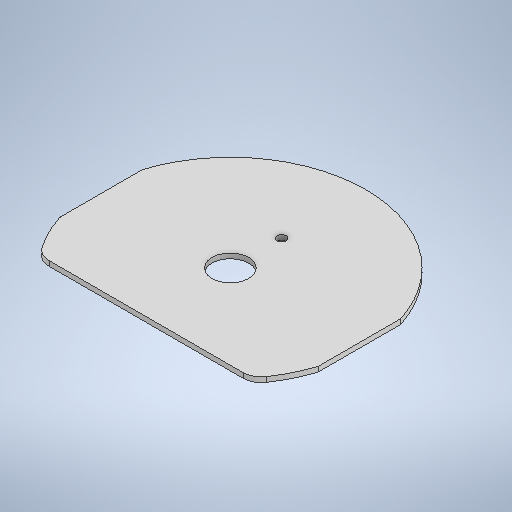
# Autodesk Inventor part: tapa_carcasa_4.0
Saved by Autodesk Inventor 2025.3 (Build 293356030, 356C)
## iProperties
Created: 2025-10-09
Part Number: tapa_carcasa_4.0
Material: Generic
Document SubType Name: Modeling
Designer: brene
Density: 1 g/cm^3
Appearance: Default
Author: brene
Autodesk Inventor part; units mm, degrees
ref_plane "YZ Plane" through (0, 0, 0) normal (1, 0, 0) x (0, 1, 0)
ref_plane "XZ Plane" through (0, 0, 0) normal (0, 1, 0) x (-1, 0, 0)
ref_plane "XY Plane" through (0, 0, 0) normal (0, 0, 1) x (1, 0, 0)
sketch "Sketch3" plane through (0, 0, 0) normal (0, 1, 0) x (-1, 0, 0)
  line L0 (0, 0) -> (67.5, 0)
  line L1 (0, 0) -> (0, 46)
  line L2 (70.5, 22.4889) -> (70.5, -22.4889)
  line L3 (0, 46) -> (52.915, 46)
  line L4 (-70.5, 22.4889) -> (-70.5, -22.4889)
  line L5 (0, 46) -> (-52.915, 46)
  arc A0 (70.5, 22.4889) -> (61.183, 41.625) centre (0, 0) ccw
  arc A1 (-61.183, 41.625) -> (-70.5, 22.4889) centre (0, 0) ccw
  arc A2 (-70.5, -22.4889) -> (70.5, -22.4889) centre (0, 0) ccw
  arc A3 (61.183, 41.625) -> (52.915, 46) centre (52.915, 36) ccw
  arc A4 (-52.915, 46) -> (-61.183, 41.625) centre (-52.915, 36) ccw
  point P0 (57.9655, 46)
  point P1 (-57.9655, 46)
  dimension "d28" = 67.5
  dimension "d29" = 46
  dimension "d30" = 10
  dimension "d31" = 10
  dimension "d32" = 74
  dimension "d34" = 70.5
  dimension "d35" = 74
  constraints: 12 end point, 12 point on circle, 5 centre point, 4 tangent, 3 symmetric about line, 2 horizontal, 2 point on line, 1 perpendicular, 1 vertical
  measures "d28" distance of L0.start L0.end
  measures "d29" distance of L0.start L1.end
  measures "d30" radius of A3
  measures "d31" radius of A4
  measures "d32" radius of A2
  measures "d34" distance between parallel lines of L2 L1
  measures "d35" radius of A1
extrude "Extrusion2" add sketch "Sketch3" along normal blind 2.7
sketch "Sketch4" plane through (0, 2.7, 0) normal (0, 1, 0) x (1, 0, 0)
  line L0 (-52.915, -46) -> (52.915, -46) projected
  line L1 (0, -46) -> (0, 0)
  circle A0 centre (0, 0) radius 10
  arc A1 (70.5, 22.4889) -> (-70.5, 22.4889) centre (0, 0) ccw projected
  line L2 (0, 74) -> (0, 28)
  circle A2 centre (0, 28) radius 2.5
  dimension "d36" = 20
  dimension "d37" = 46
  dimension "d38" = 5
  constraints: 4 end point, 2 centre point, 2 coincident, 2 vertical, 1 midpoint, 1 point on circle
  measures "d36" diameter of A0
  measures "d37" distance of L2.start L2.end
  measures "d38" diameter of A2
extrude "Extrusion3" cut sketch "Sketch4" against normal blind 10
body "Solid2"
